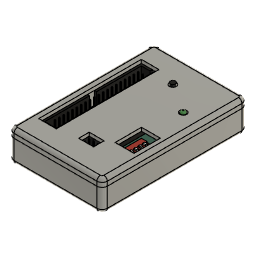
PETDiag_Clip v4 (Autodesk Fusion 360 design; units mm, degrees)
Autodesk Fusion 360 part; units mm, degrees
note: some values were not read from the file. Set by a fixed rule: which sketch regions a step uses.
(part 1 of 2)
sketch "dxf" plane through (0, 0, 0) normal (0, 0, 1) x (1, 0, 0) in component "PCB"
  line L0 (47, 0) -> (47, 77)
  line L1 (0, 77) -> (0, 0)
  line L2 (0, 0) -> (47, 0)
  line L3 (47, 77) -> (0, 77)
  line L4 (43.3388, 35.4013) -> (43.0213, 35.0838)
  line L5 (38.8938, 35.4013) -> (43.3388, 35.4013)
  line L6 (38.8938, 35.4013) -> (39.2112, 35.0838)
  line L7 (38.8938, 35.4013) -> (39.2112, 35.7188)
  line L8 (43.3388, 35.4013) -> (43.0213, 35.7188)
  line L9 (20.9118, 60.9092) -> (21.4311, 60.9092)
  arc A0 (22.4081, 60.8118) -> (22.116, 60.9092) centre (22.116, 60.4224) ccw
  line L10 (21.4311, 59.7408) -> (20.9118, 59.7408)
  line L11 (23.8432, 60.9092) -> (24.4923, 60.9092)
  line L12 (23.4885, 59.7408) -> (22.9692, 59.7408)
  line L13 (22.9692, 60.3899) -> (23.3587, 60.3899)
  arc A1 (22.2134, 59.7408) -> (22.473, 60.0004) centre (22.2134, 60.0004) ccw
  line L14 (22.9692, 59.7408) -> (22.9692, 60.9092)
  arc A2 (21.8564, 60.6496) -> (21.9862, 60.4224) centre (22.1201, 60.6496) ccw
  line L15 (19.685, 61.1124) -> (24.5431, 61.1124)
  line L16 (19.7358, 59.7408) -> (19.7358, 60.9092)
  arc A3 (21.8239, 59.9031) -> (22.2134, 59.7408) centre (22.2134, 60.2893) ccw
  arc A4 (22.473, 60.0004) -> (22.3432, 60.2276) centre (22.2093, 60.0004) ccw
  arc A5 (22.116, 60.9092) -> (21.8564, 60.6496) centre (22.116, 60.6496) ccw
  line L17 (19.7358, 60.9092) -> (20.0604, 60.9092)
  line L18 (24.1678, 59.7408) -> (24.1678, 60.9092)
  line L19 (22.9692, 60.9092) -> (23.4885, 60.9092)
  line L20 (20.9118, 59.7408) -> (20.9118, 60.9092)
  arc A6 (20.0604, 60.26) -> (20.0604, 60.9092) centre (20.0604, 60.5846) ccw
  line L21 (20.0604, 60.2601) -> (19.7358, 60.2601)
  line L22 (20.9118, 60.3899) -> (21.3013, 60.3899)
  line L23 (22.3432, 60.2276) -> (21.9862, 60.4224)
  line L24 (20.3849, 59.7408) -> (20.1253, 60.2601)
  line L25 (38.0492, 35.9855) -> (38.0492, 34.8171)
  line L26 (44.0246, 34.8171) -> (44.5438, 34.8171)
  line L27 (37.4001, 34.8171) -> (37.4001, 35.9855)
  line L28 (44.0246, 35.9855) -> (44.0246, 34.8171)
  line L29 (37.4001, 35.4662) -> (38.0492, 35.4662)
  line L30 (1.7462, 63.1975) -> (1.7462, 63.3563)
  arc A7 (16.383, 5.334) -> (16.383, 7.366) centre (16.383, 6.35) ccw
  arc A8 (23.3363, 18.542) -> (20.7963, 18.542) centre (22.0663, 18.542) ccw
  circle A9 centre (5, 72) radius 3.1789
  line L31 (1.7462, 63.3563) -> (1.7462, 63.515)
  line L32 (1.7462, 40.8138) -> (1.7462, 62.0863)
  line L33 (1.7462, 63.6738) -> (1.7462, 67.96)
  line L34 (28.6703, 53.848) -> (15.4623, 53.848)
  line L35 (1.7462, 62.0863) -> (1.7462, 62.4038)
  line L36 (8.0963, 67.96) -> (9.525, 67.96)
  line L37 (1.7462, 63.515) -> (1.7462, 63.6738)
  line L38 (10.9538, 9.54) -> (9.525, 9.54)
  line L39 (23.3362, 18.542) -> (28.6703, 18.542)
  circle A10 centre (5, 5) radius 3.1789
  line L40 (15.4623, 18.542) -> (15.4623, 53.848)
  line L41 (1.7462, 67.96) -> (8.0963, 67.96)
  line L42 (16.383, 3.302) -> (35.687, 3.302)
  line L43 (1.7462, 62.88) -> (1.7462, 63.0388)
  line L44 (9.525, 9.54) -> (8.0963, 9.54)
  line L45 (1.7462, 62.7213) -> (1.7462, 62.88)
  line L46 (35.687, 9.398) -> (16.383, 9.398)
  line L47 (8.0963, 10.3337) -> (8.0963, 9.54)
  line L48 (2.54, 40.8138) -> (1.7462, 40.8138)
  line L49 (10.16, 67.1663) -> (10.16, 10.3337)
  line L50 (1.7462, 9.54) -> (1.7462, 36.6862)
  line L51 (3.0162, 10.81) -> (2.54, 10.3337)
  line L52 (28.6703, 18.542) -> (28.6703, 53.848)
  line L53 (7.366, 62.626) -> (7.874, 62.626)
  line L54 (8.0963, 10.3337) -> (2.54, 10.3337)
  line L55 (9.525, 66.69) -> (9.6838, 66.69)
  line L56 (9.525, 10.81) -> (8.0963, 10.81)
  line L57 (3.0162, 40.8138) -> (3.0162, 66.69)
  line L58 (1.7462, 36.6862) -> (1.7462, 40.8138)
  line L59 (8.0963, 66.69) -> (8.0963, 67.1663)
  arc A11 (10.9538, 38.2738) -> (10.9538, 39.385) centre (10.9538, 38.8294) ccw
  line L60 (15.4623, 18.542) -> (20.7963, 18.542)
  line L61 (1.7462, 62.5625) -> (1.7462, 62.7213)
  line L62 (1.7462, 63.1975) -> (1.7462, 63.0388)
  line L63 (2.54, 36.6862) -> (1.7462, 36.6862)
  line L64 (9.6838, 10.81) -> (9.525, 10.81)
  line L65 (8.0963, 9.54) -> (1.7462, 9.54)
  line L66 (3.0162, 36.6862) -> (2.54, 36.6862)
  line L67 (9.6838, 66.69) -> (9.6838, 10.81)
  line L68 (3.0162, 10.81) -> (3.0162, 36.6862)
  line L69 (1.7462, 62.5625) -> (1.7463, 62.5625)
  line L70 (8.0963, 10.81) -> (3.0162, 10.81)
  circle A12 centre (5, 5) radius 1.7463
  circle A13 centre (42, 72) radius 1.7463
  line L71 (35.687, 9.398) -> (35.687, 3.302)
  line L72 (9.525, 10.3337) -> (10.16, 10.3337)
  line L73 (16.383, 9.398) -> (16.383, 7.366)
  circle A14 centre (42, 5) radius 1.7463
  line L74 (4.826, 62.626) -> (5.334, 62.626)
  line L75 (9.525, 10.81) -> (9.525, 10.3337)
  line L76 (9.525, 66.69) -> (9.525, 67.1663)
  line L77 (16.383, 3.302) -> (16.383, 5.334)
  arc A15 (10.9538, 65.42) -> (10.9538, 66.69) centre (10.9538, 66.055) ccw
  line L78 (8.0963, 67.1663) -> (8.0963, 67.96)
  line L79 (9.525, 10.3337) -> (9.525, 9.54)
  line L80 (5.334, 62.626) -> (5.334, 63.134)
  line L81 (9.525, 67.1663) -> (9.525, 67.96)
  line L82 (3.0162, 66.69) -> (8.0963, 66.69)
  line L83 (10.16, 67.1663) -> (9.6838, 66.69)
  line L84 (1.7462, 62.4038) -> (1.7462, 62.5625)
  line L85 (10.9538, 67.96) -> (10.9538, 9.54)
  circle A16 centre (5, 72) radius 1.7463
  line L86 (2.2225, 62.7213) -> (2.2224, 62.7213)
  line L87 (10.16, 67.1663) -> (9.525, 67.1663)
  circle A17 centre (42, 72) radius 3.1789
  line L88 (2.54, 62.88) -> (2.5399, 62.88)
  line L89 (8.0963, 67.1663) -> (2.54, 67.1663)
  circle A18 centre (42, 5) radius 3.1789
  line L90 (5.334, 55.006) -> (5.334, 55.514)
  line L91 (7.366, 57.546) -> (7.874, 57.546)
  line L92 (7.366, 52.974) -> (7.366, 52.466)
  line L93 (7.874, 52.466) -> (7.874, 52.974)
  line L94 (4.826, 58.054) -> (4.826, 57.546)
  line L95 (5.334, 55.514) -> (4.826, 55.514)
  line L96 (5.334, 60.086) -> (5.334, 60.594)
  line L97 (4.826, 57.546) -> (5.334, 57.546)
  line L98 (7.874, 60.594) -> (7.366, 60.594)
  line L99 (4.826, 63.134) -> (4.826, 62.626)
  line L100 (7.874, 63.134) -> (7.366, 63.134)
  line L101 (7.366, 52.466) -> (7.874, 52.466)
  line L102 (7.874, 55.514) -> (7.366, 55.514)
  line L103 (4.826, 55.514) -> (4.826, 55.006)
  line L104 (4.826, 60.086) -> (5.334, 60.086)
  line L105 (2.54, 36.6862) -> (2.54, 10.3337)
  line L106 (4.826, 49.926) -> (5.334, 49.926)
  line L107 (7.874, 49.926) -> (7.874, 50.434)
  line L108 (4.826, 52.466) -> (5.334, 52.466)
  line L109 (7.366, 58.054) -> (7.366, 57.546)
  line L110 (7.874, 52.974) -> (7.366, 52.974)
  line L111 (3.0162, 36.6862) -> (3.0162, 40.8138)
  line L112 (9.6838, 10.81) -> (10.16, 10.3337)
  line L113 (5.334, 47.894) -> (4.826, 47.894)
  line L114 (7.366, 49.926) -> (7.874, 49.926)
  line L115 (9.525, 67.96) -> (10.9538, 67.96)
  line L116 (2.54, 62.88) -> (2.54, 67.1663)
  line L117 (7.366, 50.434) -> (7.366, 49.926)
  line L118 (5.334, 52.974) -> (4.826, 52.974)
  line L119 (7.366, 44.846) -> (7.874, 44.846)
  line L120 (7.874, 57.546) -> (7.874, 58.054)
  line L121 (2.54, 40.8138) -> (2.54, 62.88)
  line L122 (4.826, 60.594) -> (4.826, 60.086)
  line L123 (7.874, 55.006) -> (7.874, 55.514)
  line L124 (7.366, 55.514) -> (7.366, 55.006)
  line L125 (4.826, 50.434) -> (4.826, 49.926)
  line L126 (7.874, 50.434) -> (7.366, 50.434)
  line L127 (5.334, 50.434) -> (4.826, 50.434)
  line L128 (5.334, 58.054) -> (4.826, 58.054)
  line L129 (7.366, 45.354) -> (7.366, 44.846)
  arc A19 (10.9538, 10.81) -> (10.9538, 12.08) centre (10.9538, 11.445) ccw
  line L130 (5.334, 49.926) -> (5.334, 50.434)
  line L131 (4.826, 47.386) -> (5.334, 47.386)
  line L132 (5.334, 47.386) -> (5.334, 47.894)
  line L133 (4.826, 55.006) -> (5.334, 55.006)
  line L134 (7.366, 60.594) -> (7.366, 60.086)
  line L135 (3.0162, 40.8138) -> (2.54, 40.8138)
  line L136 (5.334, 63.134) -> (4.826, 63.134)
  line L137 (8.0963, 10.81) -> (8.0963, 10.3337)
  line L138 (7.874, 62.626) -> (7.874, 63.134)
  line L139 (2.54, 67.1663) -> (3.0162, 66.69)
  line L140 (8.0963, 66.69) -> (9.525, 66.69)
  line L141 (7.874, 60.086) -> (7.874, 60.594)
  line L142 (7.366, 63.134) -> (7.366, 62.626)
  line L143 (7.366, 47.386) -> (7.874, 47.386)
  line L144 (5.334, 60.594) -> (4.826, 60.594)
  line L145 (5.334, 52.466) -> (5.334, 52.974)
  line L146 (7.874, 47.894) -> (7.366, 47.894)
  line L147 (7.874, 47.386) -> (7.874, 47.894)
  line L148 (4.826, 47.894) -> (4.826, 47.386)
  line L149 (7.874, 58.054) -> (7.366, 58.054)
  line L150 (7.366, 34.686) -> (7.874, 34.686)
  line L151 (7.366, 32.654) -> (7.366, 32.146)
  line L152 (4.826, 32.654) -> (4.826, 32.146)
  line L153 (7.874, 32.654) -> (7.366, 32.654)
  line L154 (7.366, 47.894) -> (7.366, 47.386)
  line L155 (7.366, 37.734) -> (7.366, 37.226)
  line L156 (4.826, 39.766) -> (5.334, 39.766)
  line L157 (5.334, 45.354) -> (4.826, 45.354)
  line L158 (7.874, 40.274) -> (7.366, 40.274)
  line L159 (7.874, 30.114) -> (7.366, 30.114)
  line L160 (7.874, 42.306) -> (7.874, 42.814)
  line L161 (7.366, 60.086) -> (7.874, 60.086)
  line L162 (7.874, 42.814) -> (7.366, 42.814)
  line L163 (5.334, 32.654) -> (4.826, 32.654)
  line L164 (5.334, 37.734) -> (4.826, 37.734)
  line L165 (5.334, 42.814) -> (4.826, 42.814)
  line L166 (5.334, 40.274) -> (4.826, 40.274)
  line L167 (7.366, 55.006) -> (7.874, 55.006)
  line L168 (4.826, 42.814) -> (4.826, 42.306)
  line L169 (5.334, 42.306) -> (5.334, 42.814)
  line L170 (7.874, 44.846) -> (7.874, 45.354)
  line L171 (7.874, 32.146) -> (7.874, 32.654)
  line L172 (7.874, 45.354) -> (7.366, 45.354)
  line L173 (7.874, 34.686) -> (7.874, 35.194)
  line L174 (5.334, 39.766) -> (5.334, 40.274)
  line L175 (4.826, 44.846) -> (5.334, 44.846)
  line L176 (7.366, 35.194) -> (7.366, 34.686)
  line L177 (4.826, 40.274) -> (4.826, 39.766)
  line L178 (7.366, 32.146) -> (7.874, 32.146)
  line L179 (5.334, 25.034) -> (4.826, 25.034)
  line L180 (4.826, 19.446) -> (5.334, 19.446)
  line L181 (4.826, 32.146) -> (5.334, 32.146)
  line L182 (5.334, 29.606) -> (5.334, 30.114)
  line L183 (5.334, 19.954) -> (4.826, 19.954)
  line L184 (4.826, 25.034) -> (4.826, 24.526)
  line L185 (4.826, 34.686) -> (5.334, 34.686)
  line L186 (4.826, 35.194) -> (4.826, 34.686)
  line L187 (4.826, 37.226) -> (5.334, 37.226)
  line L188 (7.874, 37.226) -> (7.874, 37.734)
  line L189 (4.826, 45.354) -> (4.826, 44.846)
  line L190 (7.874, 29.606) -> (7.874, 30.114)
  line L191 (7.366, 37.226) -> (7.874, 37.226)
  line L192 (7.366, 42.306) -> (7.874, 42.306)
  line L193 (7.874, 39.766) -> (7.874, 40.274)
  line L194 (7.366, 29.606) -> (7.874, 29.606)
  line L195 (5.334, 37.226) -> (5.334, 37.734)
  line L196 (7.366, 40.274) -> (7.366, 39.766)
  line L197 (4.826, 19.954) -> (4.826, 19.446)
  line L198 (4.826, 21.986) -> (5.334, 21.986)
  line L199 (7.366, 30.114) -> (7.366, 29.606)
  line L200 (5.334, 27.574) -> (4.826, 27.574)
  line L201 (5.334, 57.546) -> (5.334, 58.054)
  line L202 (4.826, 52.974) -> (4.826, 52.466)
  line L203 (5.334, 32.146) -> (5.334, 32.654)
  line L204 (7.874, 35.194) -> (7.366, 35.194)
  line L205 (5.334, 44.846) -> (5.334, 45.354)
  line L206 (7.366, 39.766) -> (7.874, 39.766)
  line L207 (7.366, 42.814) -> (7.366, 42.306)
  line L208 (4.826, 37.734) -> (4.826, 37.226)
  line L209 (7.874, 37.734) -> (7.366, 37.734)
  line L210 (4.826, 30.114) -> (4.826, 29.606)
  line L211 (5.334, 34.686) -> (5.334, 35.194)
  line L212 (4.826, 42.306) -> (5.334, 42.306)
  line L213 (5.334, 35.194) -> (4.826, 35.194)
  line L214 (5.334, 22.494) -> (4.826, 22.494)
  line L215 (34.29, 53.975) -> (33.02, 53.975)
  line L216 (28.2575, 15.7163) -> (28.2575, 11.9063)
  line L217 (34.29, 48.895) -> (33.02, 48.895)
  line L218 (25.0825, 11.2713) -> (25.7175, 11.9063)
  line L219 (30.7975, 15.7163) -> (30.7975, 11.9063)
  line L220 (7.874, 19.954) -> (7.366, 19.954)
  line L221 (5.334, 21.986) -> (5.334, 22.494)
  line L222 (23.8125, 16.3513) -> (25.0825, 16.3513)
  line L223 (7.366, 25.034) -> (7.366, 24.526)
  line L224 (5.334, 19.446) -> (5.334, 19.954)
  line L225 (7.366, 16.906) -> (7.874, 16.906)
  line L226 (26.3525, 11.2713) -> (27.6225, 11.2713)
  line L227 (25.7175, 15.7163) -> (25.7175, 11.9063)
  line L228 (5.334, 16.906) -> (5.334, 17.414)
  line L229 (4.826, 17.414) -> (4.826, 16.906)
  line L230 (26.3525, 16.3513) -> (27.6225, 16.3513)
  line L231 (28.2575, 15.7163) -> (28.8925, 16.3513)
  line L232 (7.874, 24.526) -> (7.874, 25.034)
  line L233 (4.826, 14.874) -> (4.826, 14.366)
  line L234 (7.874, 19.446) -> (7.874, 19.954)
  line L235 (7.874, 25.034) -> (7.366, 25.034)
  line L236 (7.874, 27.066) -> (7.874, 27.574)
  line L237 (7.366, 27.574) -> (7.366, 27.066)
  line L238 (7.874, 27.574) -> (7.366, 27.574)
  line L239 (23.1775, 11.9063) -> (23.1775, 15.7163)
  line L240 (7.874, 14.874) -> (7.366, 14.874)
  line L241 (32.385, 52.07) -> (32.385, 53.975)
  line L242 (7.366, 19.446) -> (7.874, 19.446)
  line L243 (5.334, 30.114) -> (4.826, 30.114)
  line L244 (7.366, 19.954) -> (7.366, 19.446)
  line L245 (4.826, 16.906) -> (5.334, 16.906)
  line L246 (7.366, 21.986) -> (7.874, 21.986)
  line L247 (25.7175, 11.9063) -> (26.3525, 11.2713)
  line L248 (32.385, 49.53) -> (32.385, 50.8)
  line L249 (33.02, 53.975) -> (32.385, 53.975)
  line L250 (34.925, 50.8) -> (34.925, 49.53)
  line L251 (4.826, 22.494) -> (4.826, 21.986)
  line L252 (7.874, 14.366) -> (7.874, 14.874)
  line L253 (5.334, 14.366) -> (5.334, 14.874)
  line L254 (5.334, 27.066) -> (5.334, 27.574)
  line L255 (4.826, 27.066) -> (5.334, 27.066)
  line L256 (5.334, 14.874) -> (4.826, 14.874)
  line L257 (4.826, 27.574) -> (4.826, 27.066)
  line L258 (27.6225, 11.2713) -> (28.2575, 11.9063)
  line L259 (7.366, 14.874) -> (7.366, 14.366)
  line L260 (7.874, 17.414) -> (7.366, 17.414)
  line L261 (7.366, 22.494) -> (7.366, 21.986)
  line L262 (7.874, 22.494) -> (7.366, 22.494)
  line L263 (5.334, 17.414) -> (4.826, 17.414)
  line L264 (5.334, 24.526) -> (5.334, 25.034)
  line L265 (7.874, 21.986) -> (7.874, 22.494)
  line L266 (7.366, 24.526) -> (7.874, 24.526)
  line L267 (7.366, 27.066) -> (7.874, 27.066)
  line L268 (7.366, 17.414) -> (7.366, 16.906)
  line L269 (4.826, 24.526) -> (5.334, 24.526)
  line L270 (4.826, 14.366) -> (5.334, 14.366)
  line L271 (7.366, 14.366) -> (7.874, 14.366)
  line L272 (4.826, 29.606) -> (5.334, 29.606)
  line L273 (7.874, 16.906) -> (7.874, 17.414)
  line L274 (34.925, 52.07) -> (34.6075, 51.7525)
  line L275 (27.6225, 16.3513) -> (28.2575, 15.7163)
  line L276 (34.6075, 51.1175) -> (34.925, 50.8)
  line L277 (34.925, 53.34) -> (34.925, 52.07)
  circle A20 centre (23, 65) radius 1.75
  arc A21 (25.45, 63.25) -> (25.45, 62.45) centre (25.15, 62.85) ccw
  line L278 (34.925, 53.34) -> (34.29, 53.975)
  line L279 (25.7175, 15.7163) -> (26.3525, 16.3513)
  line L280 (32.7025, 51.7525) -> (32.385, 52.07)
  line L281 (30.1625, 11.2713) -> (30.7975, 11.9063)
  line L282 (45.7518, 33.9408) -> (42.4498, 33.9408)
  line L283 (26, 66.45) -> (26, 63.6)
  line L284 (23.1775, 11.9063) -> (23.1775, 11.2713)
  line L285 (30.1625, 16.3513) -> (30.7975, 15.7163)
  line L286 (25.0825, 16.3513) -> (25.7175, 15.7163)
  line L287 (28.8925, 16.3513) -> (30.1625, 16.3513)
  line L288 (32.385, 50.8) -> (32.7025, 51.1175)
  line L289 (23.1775, 11.2713) -> (25.0825, 11.2713)
  line L290 (28.8925, 11.2713) -> (30.1625, 11.2713)
  arc A22 (41.5, 54.8) -> (38.5, 54.8) centre (40, 54) ccw
  arc A23 (20.55, 62.45) -> (20.5, 63.2) centre (20.8502, 62.8467) ccw
  circle A24 centre (23, 65) radius 1.4
  line L291 (28.2575, 11.9063) -> (28.8925, 11.2713)
  line L292 (23.1775, 15.7163) -> (23.8125, 16.3513)
  line L293 (25.4, 62) -> (20.25, 62)
  line L294 (20, 63.55) -> (20, 66.45)
  arc A25 (20.55, 66.75) -> (20.5, 67.5) centre (20.8502, 67.1467) ccw
  line L295 (33.02, 48.895) -> (32.385, 49.53)
  arc A26 (41.5, 54.8) -> (38.5, 54.8) centre (40, 54) ccw
  arc A27 (38.5, 53.2) -> (41.5, 53.2) centre (40, 54) ccw
  line L296 (34.925, 49.53) -> (34.29, 48.895)
  arc A28 (38.5, 53.2) -> (41.5, 53.2) centre (40, 54) ccw
  line L297 (39.1478, 33.4327) -> (42.4498, 33.4327)
  line L298 (20.25, 68) -> (25.75, 68)
  line L299 (41.6878, 32.6707) -> (38.8938, 32.6707)
  line L300 (39.1478, 33.9408) -> (35.8458, 33.9408)
  line L301 (42.4498, 32.6707) -> (42.7037, 32.6707)
  line L302 (35.8458, 19.7168) -> (39.1478, 19.7168)
  line L303 (38.8938, 23.5267) -> (41.6878, 23.5267)
  line L304 (42.4498, 19.7168) -> (45.7518, 19.7168)
  line L305 (41.6878, 25.0508) -> (38.8938, 25.0508)
  line L306 (38.8938, 23.5267) -> (38.8938, 25.0508)
  line L307 (42.7037, 31.1468) -> (42.4498, 31.1468)
  line L308 (40.7988, 24.7968) -> (39.1478, 24.7968)
  line L309 (42.7037, 28.8608) -> (42.7037, 28.6068)
  line L310 (42.7037, 23.5267) -> (42.4498, 23.5267)
  line L311 (42.7037, 25.0508) -> (42.7037, 24.7968)
  line L312 (38.8938, 20.9868) -> (41.6878, 20.9868)
  line L313 (40.7988, 29.8768) -> (39.1478, 29.8768)
  line L314 (42.4498, 30.1308) -> (42.7037, 30.1308)
  line L315 (38.8938, 31.1468) -> (41.6878, 31.1468)
  line L316 (40.7988, 21.2408) -> (39.1478, 21.2408)
  line L317 (40.7988, 22.2568) -> (39.1478, 22.2568)
  line L318 (40.7988, 26.3208) -> (39.1478, 26.3208)
  line L319 (42.4498, 33.4327) -> (42.4498, 33.9408)
  line L320 (42.7037, 31.4008) -> (42.7037, 31.1468)
  line L321 (38.8938, 28.6068) -> (38.8938, 30.1308)
  line L322 (42.7037, 26.3208) -> (42.7037, 26.0668)
  line L323 (40.7988, 28.8608) -> (39.1478, 28.8608)
  line L324 (40.7988, 27.3368) -> (39.1478, 27.3368)
  line L325 (39.1478, 29.8768) -> (39.1478, 28.8608)
  line L326 (42.4498, 20.2248) -> (39.1478, 20.2248)
  line L327 (41.6878, 30.1308) -> (38.8938, 30.1308)
  line L328 (38.8938, 28.6068) -> (41.6878, 28.6068)
  line L329 (39.1478, 33.9408) -> (39.1478, 33.4327)
  line L330 (42.7037, 27.5907) -> (42.7037, 27.3368)
  line L331 (38.8938, 26.0668) -> (38.8938, 27.5907)
  line L332 (39.1478, 20.2248) -> (39.1478, 19.7168)
  line L333 (42.7037, 30.1308) -> (42.7037, 29.8768)
  arc A29 (25.45, 67.55) -> (25.5, 66.8) centre (25.1498, 67.1533) ccw
  line L334 (42.7037, 32.6707) -> (42.7037, 32.4168)
  line L335 (39.1478, 19.7168) -> (42.4498, 19.7168)
  line L336 (35.8458, 33.9408) -> (35.8458, 19.7168)
  line L337 (40.7988, 32.4168) -> (39.1478, 32.4168)
  line L338 (42.4498, 27.5907) -> (42.7037, 27.5907)
  line L339 (42.7037, 23.7808) -> (42.7037, 23.5267)
  line L340 (42.4498, 19.7168) -> (42.4498, 20.2248)
  line L341 (41.6878, 22.5108) -> (38.8938, 22.5108)
  line L342 (40.7988, 31.4008) -> (39.1478, 31.4008)
  line L343 (41.6878, 27.5907) -> (38.8938, 27.5907)
  line L344 (38.8938, 20.9868) -> (38.8938, 22.5108)
  line L345 (38.8938, 31.1468) -> (38.8938, 32.6707)
  line L346 (42.4498, 25.0508) -> (42.7037, 25.0508)
  line L347 (45.7518, 19.7168) -> (45.7518, 33.9408)
  line L348 (42.7037, 28.6068) -> (42.4498, 28.6068)
  line L349 (38.8938, 26.0668) -> (41.6878, 26.0668)
  line L350 (42.4498, 33.9408) -> (39.1478, 33.9408)
  line L351 (42.7037, 26.0668) -> (42.4498, 26.0668)
  line L352 (40.7988, 23.7808) -> (39.1478, 23.7808)
  line L353 (40.7988, 22.2568) -> (40.4178, 22.2568)
  line L354 (39.7828, 27.3368) -> (39.7828, 26.3208)
  line L355 (40.7988, 28.8608) -> (40.7988, 29.8768)
  line L356 (40.7988, 31.4008) -> (40.7988, 32.4168)
  line L357 (39.5288, 32.4168) -> (39.1478, 32.4168)
  line L358 (39.5288, 21.2408) -> (39.5288, 22.2568)
  line L359 (39.1478, 26.3208) -> (39.5288, 26.3208)
  line L360 (40.4178, 23.7808) -> (40.7988, 23.7808)
  line L361 (39.1478, 23.7808) -> (39.5288, 23.7808)
  line L362 (39.7828, 32.4168) -> (39.7828, 31.4008)
  line L363 (40.4178, 24.7968) -> (40.4178, 23.7808)
  line L364 (39.5288, 23.7808) -> (39.5288, 24.7968)
  line L365 (39.1478, 31.4008) -> (39.5288, 31.4008)
  line L366 (39.5288, 26.3208) -> (39.5288, 27.3368)
  line L367 (39.7828, 21.2408) -> (40.1638, 21.2408)
  line L368 (39.7828, 26.3208) -> (40.1638, 26.3208)
  line L369 (40.1638, 23.7808) -> (40.1638, 24.7968)
  line L370 (39.1478, 22.2568) -> (39.1478, 21.2408)
  line L371 (40.4178, 28.8608) -> (40.7988, 28.8608)
  line L372 (42.7037, 20.9868) -> (42.4498, 20.9868)
  line L373 (40.4178, 22.2568) -> (40.4178, 21.2408)
  line L374 (40.1638, 27.3368) -> (39.7828, 27.3368)
  line L375 (39.7828, 23.7808) -> (40.1638, 23.7808)
  line L376 (39.7828, 28.8608) -> (40.1638, 28.8608)
  line L377 (39.1478, 24.7968) -> (39.1478, 23.7808)
  line L378 (39.1478, 21.2408) -> (39.5288, 21.2408)
  line L379 (40.1638, 22.2568) -> (39.7828, 22.2568)
  line L380 (42.7037, 22.5108) -> (42.7037, 22.2568)
  line L381 (40.4178, 29.8768) -> (40.4178, 28.8608)
  line L382 (39.5288, 22.2568) -> (39.1478, 22.2568)
  line L383 (40.7988, 32.4168) -> (40.4178, 32.4168)
  line L384 (40.7988, 21.2408) -> (40.7988, 22.2568)
  line L385 (39.5288, 31.4008) -> (39.5288, 32.4168)
  line L386 (40.7988, 23.7808) -> (40.7988, 24.7968)
  line L387 (40.4178, 21.2408) -> (40.7988, 21.2408)
  line L388 (40.1638, 29.8768) -> (39.7828, 29.8768)
  line L389 (40.7988, 26.3208) -> (40.7988, 27.3368)
  line L390 (39.7828, 31.4008) -> (40.1638, 31.4008)
  line L391 (40.4178, 32.4168) -> (40.4178, 31.4008)
  line L392 (40.1638, 21.2408) -> (40.1638, 22.2568)
  line L393 (40.1638, 31.4008) -> (40.1638, 32.4168)
  line L394 (40.4178, 31.4008) -> (40.7988, 31.4008)
  line L395 (40.1638, 32.4168) -> (39.7828, 32.4168)
  line L396 (40.7988, 27.3368) -> (40.4178, 27.3368)
  line L397 (39.7828, 29.8768) -> (39.7828, 28.8608)
  line L398 (39.5288, 28.8608) -> (39.5288, 29.8768)
  line L399 (39.1478, 27.3368) -> (39.1478, 26.3208)
  line L400 (39.1478, 28.8608) -> (39.5288, 28.8608)
  line L401 (40.1638, 28.8608) -> (40.1638, 29.8768)
  line L402 (39.5288, 24.7968) -> (39.1478, 24.7968)
  line L403 (42.7037, 21.2408) -> (42.7037, 20.9868)
  line L404 (39.5288, 27.3368) -> (39.1478, 27.3368)
  line L405 (39.1478, 32.4168) -> (39.1478, 31.4008)
  line L406 (42.4498, 22.5108) -> (42.7037, 22.5108)
  line L407 (40.7988, 29.8768) -> (40.4178, 29.8768)
  line L408 (39.7828, 22.2568) -> (39.7828, 21.2408)
  line L409 (40.4178, 26.3208) -> (40.7988, 26.3208)
  line L410 (40.4178, 27.3368) -> (40.4178, 26.3208)
  line L411 (40.7988, 24.7968) -> (40.4178, 24.7968)
  line L412 (39.7828, 24.7968) -> (39.7828, 23.7808)
  line L413 (40.1638, 26.3208) -> (40.1638, 27.3368)
  line L414 (40.1638, 24.7968) -> (39.7828, 24.7968)
  line L415 (39.5288, 29.8768) -> (39.1478, 29.8768)
  line L416 (24.7015, 12.2872) -> (24.7015, 12.7952)
  line L417 (24.7015, 12.7952) -> (24.1935, 12.7952)
  line L418 (33.401, 52.959) -> (33.401, 52.451)
  line L419 (34.6075, 51.7525) -> (34.29, 51.435)
  line L420 (34.29, 51.435) -> (33.02, 51.435)
  line L421 (24.1935, 12.7952) -> (24.1935, 12.2872)
  line L422 (33.909, 52.451) -> (33.909, 52.959)
  line L423 (24.7015, 14.8273) -> (24.7015, 15.3353)
  line L424 (26.7335, 12.2872) -> (27.2415, 12.2872)
  line L425 (29.2735, 15.3353) -> (29.2735, 14.8273)
  line L426 (33.909, 52.959) -> (33.401, 52.959)
  line L427 (26.7335, 12.7952) -> (26.7335, 12.2872)
  line L428 (29.7815, 12.2872) -> (29.7815, 12.7952)
  line L429 (32.7025, 51.1175) -> (33.02, 51.435)
  line L430 (33.401, 50.419) -> (33.401, 49.911)
  line L431 (33.909, 50.419) -> (33.401, 50.419)
  line L432 (33.02, 51.435) -> (32.7025, 51.7525)
  line L433 (34.29, 51.435) -> (34.6075, 51.1175)
  line L434 (33.401, 52.451) -> (33.909, 52.451)
  line L435 (33.909, 49.911) -> (33.909, 50.419)
  line L436 (33.401, 49.911) -> (33.909, 49.911)
  line L437 (24.1935, 12.2872) -> (24.7015, 12.2872)
  line L438 (27.2415, 14.8273) -> (27.2415, 15.3353)
  line L439 (25.75, 68) -> (25.8, 68)
  line L440 (20, 63.1) -> (19.5, 63.1)
  line L441 (19.5, 63.1) -> (19.5, 62.4)
  line L442 (26.5, 63.1) -> (26, 63.1)
  arc A30 (25.5, 66.8) -> (25.45, 67.55) centre (25.1498, 67.1533) ccw
  line L443 (26, 67.8) -> (26, 66.45)
  line L444 (26, 63.1) -> (26, 62.4)
  arc A31 (25.45, 62.45) -> (25.45, 63.25) centre (25.15, 62.85) ccw
  line L445 (26, 67.6) -> (26, 66.9)
  line L446 (20, 62.2) -> (20, 63.55)
  line L447 (25.8, 62) -> (25.4, 62)
  line L448 (26, 66.9) -> (26.5, 66.9)
  arc A32 (20.5, 63.2) -> (20.55, 62.45) centre (20.8502, 62.8467) ccw
  arc A33 (20.2, 68) -> (20, 67.8) centre (20.2, 67.8) ccw
  arc A34 (20, 62.2) -> (20.2, 62) centre (20.2, 62.2) ccw
  line L449 (29.7815, 12.7952) -> (29.2735, 12.7952)
  line L450 (19.5, 66.9) -> (20, 66.9)
  line L451 (26, 62.4) -> (26.5, 62.4)
  line L452 (26.5, 62.4) -> (26.5, 63.1)
  arc A35 (20.5, 67.5) -> (20.55, 66.75) centre (20.8502, 67.1467) ccw
  line L453 (27.2415, 12.2872) -> (27.2415, 12.7952)
  line L454 (24.7015, 15.3353) -> (24.1935, 15.3353)
  line L455 (19.5, 62.4) -> (20, 62.4)
  line L456 (42.7037, 27.3368) -> (42.7037, 26.3208)
  circle A36 centre (40, 54) radius 1.5
  line L457 (29.2735, 14.8273) -> (29.7815, 14.8273)
  line L458 (42.4498, 28.6068) -> (41.6878, 28.6068)
  line L459 (20, 66.9) -> (20, 67.6)
  line L460 (42.7037, 24.7968) -> (42.7037, 23.7808)
  line L461 (20.25, 62) -> (20.2, 62)
  line L462 (42.4498, 30.1308) -> (41.6878, 30.1308)
  line L463 (20, 66.45) -> (20, 67.8)
  line L464 (26.5, 67.6) -> (26, 67.6)
  line L465 (42.4498, 31.1468) -> (41.6878, 31.1468)
  line L466 (19.5, 67.6) -> (19.5, 66.9)
  line L467 (42.4498, 23.5267) -> (41.6878, 23.5267)
  line L468 (42.4498, 27.5907) -> (41.6878, 27.5907)
  arc A37 (41.5, 53.2) -> (41.5, 54.8) centre (40, 54) ccw
  line L469 (27.2415, 12.7952) -> (26.7335, 12.7952)
  line L470 (29.7815, 14.8273) -> (29.7815, 15.3353)
  line L471 (26.7335, 15.3353) -> (26.7335, 14.8273)
  line L472 (29.2735, 12.7952) -> (29.2735, 12.2872)
  line L473 (20, 62.4) -> (20, 63.1)
  line L474 (20, 67.6) -> (19.5, 67.6)
  line L475 (26, 63.6) -> (26, 62.2)
  arc A38 (25.8, 62) -> (26, 62.2) centre (25.8, 62.2) ccw
  line L476 (24.1935, 15.3353) -> (24.1935, 14.8273)
  line L477 (26.7335, 14.8273) -> (27.2415, 14.8273)
  line L478 (29.2735, 12.2872) -> (29.7815, 12.2872)
  line L479 (27.2415, 15.3353) -> (26.7335, 15.3353)
  line L480 (29.7815, 15.3353) -> (29.2735, 15.3353)
  line L481 (20.2, 68) -> (20.25, 68)
  line L482 (26.5, 66.9) -> (26.5, 67.6)
  line L483 (24.1935, 14.8273) -> (24.7015, 14.8273)
  line L484 (38.5, 53.2) -> (38.5, 54.8)
  arc A39 (26, 67.8) -> (25.8, 68) centre (25.8, 67.8) ccw
  line L485 (36.6713, 21.4171) -> (36.6713, 22.1933)
  line L486 (37.7578, 23.9571) -> (37.7578, 24.7333)
  line L487 (42.4498, 20.9868) -> (41.6878, 20.9868)
  line L488 (37.4474, 24.5004) -> (38.0682, 24.5004)
  line L489 (38.0682, 29.0371) -> (38.0682, 29.8133)
  arc A40 (37.6026, 22.1932) -> (37.2922, 21.8828) centre (37.6026, 21.8828) ccw
  line L490 (43.7903, 31.7008) -> (44.4112, 31.7008)
  line L491 (42.4498, 25.0508) -> (41.6878, 25.0508)
  line L492 (36.9817, 31.3231) -> (36.6713, 31.7112)
  arc A41 (37.2921, 29.6968) -> (37.0205, 29.8132) centre (37.0205, 29.4381) ccw
  line L493 (37.2921, 26.9628) -> (37.2921, 26.6524)
  line L494 (36.6713, 24.2676) -> (37.7578, 23.9571)
  line L495 (43.4023, 32.3391) -> (44.7993, 33.1153)
  line L496 (42.4498, 26.0668) -> (41.6878, 26.0668)
  line L497 (37.2921, 21.8828) -> (37.2921, 21.4171)
  line L498 (42.7037, 29.8768) -> (42.7037, 28.8608)
  line L499 (37.7578, 22.1933) -> (37.6026, 22.1933)
  line L500 (38.0682, 31.3231) -> (38.0682, 32.0993)
  line L501 (38.0682, 26.4971) -> (38.0682, 26.8852)
  line L502 (42.4498, 32.6707) -> (41.6878, 32.6707)
  arc A42 (37.2921, 26.9628) -> (36.6713, 26.9628) centre (36.9817, 26.9628) ccw
  line L503 (38.0682, 21.4171) -> (38.0682, 21.8828)
  line L504 (42.7037, 22.2568) -> (42.7037, 21.2408)
  arc A43 (44.4112, 30.9246) -> (44.4112, 31.7008) centre (44.4112, 31.3127) ccw
  line L505 (44.4112, 30.9247) -> (43.7903, 30.9247)
  line L506 (36.6713, 26.4971) -> (36.6713, 26.9628)
  line L507 (42.4498, 22.5108) -> (41.6878, 22.5108)
  arc A44 (38.0682, 21.8828) -> (37.7578, 22.1932) centre (37.7578, 21.8828) ccw
  line L508 (37.2921, 29.6968) -> (38.0682, 29.0371)
  line L509 (37.2921, 21.4171) -> (36.6713, 21.4171)
  line L510 (44.7993, 33.1153) -> (43.4023, 33.1153)
  line L511 (42.7037, 32.4168) -> (42.7037, 31.4008)
  arc A45 (38.0683, 26.8852) -> (37.2921, 26.8852) centre (37.6802, 26.8852) ccw
  arc A46 (37.0205, 29.8133) -> (36.6712, 29.464) centre (37.0205, 29.464) ccw
  line L512 (44.7993, 32.3391) -> (43.4023, 32.3391)
  line L513 (36.6713, 31.7112) -> (38.0682, 31.7112)
  arc A47 (36.6712, 29.464) -> (36.9817, 29.0371) centre (37.1199, 29.464) ccw
  arc A48 (43.7903, 31.7008) -> (43.7903, 30.9246) centre (43.7903, 31.3127) ccw
extrude "Extrude1" add sketch "dxf" against normal blind 1.6 contours L0 L1 L2 L3 | L16 L17 A6 L21 | L30 L31 L32 L33 L35 L37 L41 L43 L45 L48 L61 L62 L78 L84 L89 L116 L121 | L36 L59 L76 L78 L81 L140 | L38 L49 L72 L79 L81 L85 L87 L115 | L59 L82 L89 L139 | L55 L76 L83 L87 | L55 L56 L57 L64 L67 L68 L70 L82 L111 L140 | L57 L116 L121 L135 L139 | L48 L58 L63 L66 L111 L135 | L49 L67 L83 L112 | A15 L85 | L47 L50 L54 L63 L65 L105 | L64 L72 L75 L112 | L51 L66 L68 L105 | L44 L47 L56 L75 L79 L137 | A11 L85 | L51 L54 L70 L137 | L85 A19 | A7 L42 L46 L71 L73 L77 | A8 L34 L39 L40 L52 L60 | A9 | A10 | L53 L100 L138 L142 | L74 L80 L99 L136 | A17 | A18 | L90 L95 L103 L133 | L91 L109 L120 L149 | L92 L93 L101 L110 | L94 L97 L128 L201 | L96 L104 L122 L144 | L98 L134 L141 L161 | L102 L123 L124 L167 | L106 L125 L127 L130 | L107 L114 L117 L126 | L108 L118 L145 L202 | L113 L131 L132 L148 | L119 L129 L170 L172 | L143 L146 L147 L154 | L150 L173 L176 L204 | L151 L153 L171 L178 | L152 L163 L181 L203 | L155 L188 L191 L209 | L156 L166 L174 L177 | L157 L175 L189 L205 | L158 L193 L196 L206 | L159 L190 L194 L199 | L160 L162 L192 L207 | L164 L187 L195 L208 | L165 L168 L169 L212 | L179 L184 L264 L269 | L180 L183 L197 L224 | L182 L210 L243 L272 | L185 L186 L211 L213 | L198 L214 L221 L251 | L200 L254 L255 L257 | L215 L241 L249 L274 L277 L278 L280 L419 L420 L432 | L217 L248 L250 L276 L288 L295 L296 L420 L429 L433 | L216 L219 L231 L281 L285 L287 L290 L291 | L216 L226 L227 L230 L247 L258 L275 L279 | L218 L222 L227 L239 L284 L286 L289 L292 | L220 L234 L242 L244 | L223 L232 L235 L266 | L225 L260 L268 L273 | L228 L229 L245 L263 | L233 L253 L256 L270 | L236 L237 L238 L267 | L240 L252 L259 L271 | L246 L261 L262 L265 | A20 | A21 A31 | L282 L297 L300 L302 L304 L319 L326 L329 L332 L336 L340 L347 | L297 L319 L329 L350 | L326 L332 L335 L340 | L283 L293 L294 L298 L439 L443 L444 L445 L446 L447 A33 A34 L459 L461 L463 L473 L475 A38 L481 A39 | L443 L445 L448 L464 L482 | L442 L444 L451 L452 L475 | L450 L459 L463 L466 L474 | L440 L441 L446 L455 L473 | A36 | A22 A26 A27 A28 A37 L484 | A23 A32 | A24 | A25 A35 | L299 L301 L307 L315 L320 L334 L345 L465 L502 L511 | L303 L305 L306 L310 L311 L339 L346 L460 L467 L491 | L308 L352 L360 L363 L386 L411 | L308 L352 L363 L369 | L308 L352 L369 L375 L412 L414 | L308 L352 L364 L412 | L308 L352 L361 L364 L377 L402 | L309 L314 L321 L327 L328 L333 L348 L458 L462 L498 | L312 L341 L344 L372 L380 L403 L406 L487 L504 L507 | L313 L323 L355 L371 L381 L407 | L313 L323 L381 L401 | L313 L323 L376 L388 L397 L401 | L313 L323 L397 L398 | L313 L323 L325 L398 L400 L415 | L316 L317 L353 L373 L384 L387 | L316 L317 L373 L392 | L316 L317 L367 L379 L392 L408 | L316 L317 L358 L408 | L316 L317 L358 L370 L378 L382 | L318 L324 L389 L396 L409 L410 | L318 L324 L410 L413 | L318 L324 L354 L368 L374 L413 | L318 L324 L354 L366 | L318 L324 L359 L366 L399 L404 | L322 L330 L331 L338 L343 L349 L351 L456 L468 L496 | A29 A30 | L337 L342 L356 L383 L391 L394 | L337 L342 L391 L393 | L337 L342 L362 L390 L393 L395 | L337 L342 L362 L385 | L337 L342 L357 L365 L385 L405 | L416 L417 L421 L437 | L418 L422 L426 L434 | L423 L454 L476 L483 | L424 L427 L453 L469 | L425 L457 L470 L480 | L428 L449 L472 L478 | L430 L431 L435 L436 | L438 L471 L477 L479 | L490 A43 L505 A48 makes body 1 in component "PCB"
extrude "Extrude2" add sketch "dxf" along normal blind 9.5 contours A7 L42 L46 L71 L73 L77 | A8 L34 L39 L40 L52 L60 bodies 1 in component "PCB"
extrude "Extrude3" add sketch "dxf" along normal blind 6 contours L282 L297 L300 L302 L304 L319 L326 L329 L332 L336 L340 L347 | L490 A43 L505 A48 bodies 1 in component "PCB"
extrude "Extrude4" add sketch "dxf" along normal blind 5 contours L299 L301 L307 L315 L320 L334 L345 L465 L502 L511 | L303 L305 L306 L310 L311 L339 L346 L460 L467 L491 | L309 L314 L321 L327 L328 L333 L348 L458 L462 L498 | L312 L341 L344 L372 L380 L403 L406 L487 L504 L507 | L322 L330 L331 L338 L343 L349 L351 L456 L468 L496 bodies 1 in component "PCB"
extrude "Extrude5" add sketch "dxf" along normal blind 6.5 contours L308 L352 L360 L363 L386 L411 | L308 L352 L363 L369 | L308 L352 L369 L375 L412 L414 | L308 L352 L364 L412 | L308 L352 L361 L364 L377 L402 | L313 L323 L355 L371 L381 L407 | L313 L323 L381 L401 | L313 L323 L376 L388 L397 L401 | L313 L323 L397 L398 | L313 L323 L325 L398 L400 L415 | L316 L317 L353 L373 L384 L387 | L316 L317 L373 L392 | L316 L317 L367 L379 L392 L408 | L316 L317 L358 L408 | L316 L317 L358 L370 L378 L382 | L318 L324 L389 L396 L409 L410 | L318 L324 L410 L413 | L318 L324 L354 L368 L374 L413 | L318 L324 L354 L366 | L318 L324 L359 L366 L399 L404 | L337 L342 L356 L383 L391 L394 | L337 L342 L391 L393 | L337 L342 L362 L390 L393 L395 | L337 L342 L362 L385 | L337 L342 L357 L365 L385 L405 bodies 1 in component "PCB"
extrude "Extrude7" add sketch "dxf" along normal blind 9.5 contours L416 L417 L421 L437 | L423 L454 L476 L483 | L424 L427 L453 L469 | L425 L457 L470 L480 | L428 L449 L472 L478 | L438 L471 L477 L479 bodies 1 in component "PCB"
extrude "Extrude6" add sketch "dxf" along normal blind 2.5 contours L216 L219 L231 L281 L285 L287 L290 L291 | L216 L226 L227 L230 L247 L258 L275 L279 | L218 L222 L227 L239 L284 L286 L289 L292 bodies 1 in component "PCB"
extrude "Extrude8" add sketch "dxf" along normal blind 9.5 contours L53 L100 L138 L142 | L74 L80 L99 L136 | L90 L95 L103 L133 | L91 L109 L120 L149 | L92 L93 L101 L110 | L94 L97 L128 L201 | L96 L104 L122 L144 | L98 L134 L141 L161 | L102 L123 L124 L167 | L106 L125 L127 L130 | L107 L114 L117 L126 | L108 L118 L145 L202 | L113 L131 L132 L148 | L119 L129 L170 L172 | L143 L146 L147 L154 | L150 L173 L176 L204 | L151 L153 L171 L178 | L152 L163 L181 L203 | L155 L188 L191 L209 | L156 L166 L174 L177 | L157 L175 L189 L205 | L158 L193 L196 L206 | L159 L190 L194 L199 | L160 L162 L192 L207 | L164 L187 L195 L208 | L165 L168 L169 L212 | L179 L184 L264 L269 | L180 L183 L197 L224 | L182 L210 L243 L272 | L185 L186 L211 L213 | L198 L214 L221 L251 | L200 L254 L255 L257 | L220 L234 L242 L244 | L223 L232 L235 L266 | L225 L260 L268 L273 | L228 L229 L245 L263 | L233 L253 L256 L270 | L236 L237 L238 L267 | L240 L252 L259 L271 | L246 L261 L262 L265 bodies 1 in component "PCB"
extrude "Extrude9" add sketch "dxf" along normal blind 2 contours L36 L59 L76 L78 L81 L140 | L55 L56 L57 L64 L67 L68 L70 L82 L111 L140 | L48 L58 L63 L66 L111 L135 | L44 L47 L56 L75 L79 L137 bodies 1 in component "PCB"
extrude "Extrude10" add sketch "dxf" along normal blind 9.5 contours L30 L31 L32 L33 L35 L37 L41 L43 L45 L48 L61 L62 L78 L84 L89 L116 L121 | L38 L49 L72 L79 L81 L85 L87 L115 | L59 L82 L89 L139 | L55 L76 L83 L87 | L57 L116 L121 L135 L139 | L49 L67 L83 L112 | A15 L85 | L47 L50 L54 L63 L65 L105 | L64 L72 L75 L112 | L51 L66 L68 L105 | A11 L85 | L51 L54 L70 L137 | L85 A19 bodies 1 in component "PCB"
extrude "Extrude11" add sketch "dxf" along normal blind 12 contours A36 bodies 1 in component "PCB"
extrude "Extrude12" add sketch "dxf" along normal blind 6.3 contours A22 A26 A27 A28 A37 L484 bodies 1 in component "PCB"
fillet "Fillet1" radius 1.2 1 edges at (38.6015, 53.4576, 12) on bodies 1 in component "PCB"
extrude "Extrude13" add sketch "dxf" along normal blind 12 contours A20 | A24 bodies 1 in component "PCB"
chamfer "Chamfer1" distance 0.25 distance2 9 1 edges at (21.3684, 64.3672, 12) measured on face at (23.482, 65.5025, 12) on bodies 1 in component "PCB"
extrude "Extrude14" add sketch "dxf" along normal blind 4 contours L283 L293 L294 L298 L439 L443 L444 L445 L446 L447 A33 A34 L459 L461 L463 L473 L475 A38 L481 A39 bodies 1 in component "PCB"
extrude "Extrude15" add sketch "dxf" along normal blind 4.5 contours A21 A31 | A23 A32 | A25 A35 | A29 A30 bodies 1 in component "PCB"
ref_plane "WorkPlane1" through (23.5, 38.5, -4.6) normal (0, 0, 1) x (1, 0, 0) in component "bottom_shell"
sketch "bottom" plane through (23.5, 38.5, -4.6) normal (0, 0, 1) x (1, 0, 0) in component "bottom_shell"
  circle A0 centre (-18.5, 33.5) radius 1.7463 construction
  circle A1 centre (18.5, 33.5) radius 1.7463 construction
  circle A2 centre (18.5, -33.5) radius 1.7463 construction
  circle A3 centre (-18.5, -33.5) radius 1.7463 construction
  line L0 (23.5, -38.5) -> (23.5, 38.5) construction
  line L1 (-23.5, -38.5) -> (23.5, -38.5) construction
  line L2 (-23.5, 38.5) -> (-23.5, -38.5) construction
  line L3 (23.5, 38.5) -> (-23.5, 38.5) construction
  line L4 (25, -39) -> (25, 39)
  line L5 (24, 40) -> (-24, 40)
  line L6 (-25, 39) -> (-25, -39)
  line L7 (-24, -40) -> (24, -40)
  arc A4 (25, 39) -> (24, 40) centre (24, 39) ccw
  arc A5 (-24, 40) -> (-25, 39) centre (-24, 39) ccw
  arc A6 (24, -40) -> (25, -39) centre (24, -39) ccw
  arc A7 (-25, -39) -> (-24, -40) centre (-24, -39) ccw
  line L8 (-25.8, 39) -> (-25.8, -39)
  arc A8 (-25.8, -39) -> (-24, -40.8) centre (-24, -39) ccw
  line L9 (-24, -40.8) -> (24, -40.8)
  arc A9 (24, -40.8) -> (25.8, -39) centre (24, -39) ccw
  line L10 (25.8, -39) -> (25.8, 39)
  arc A10 (25.8, 39) -> (24, 40.8) centre (24, 39) ccw
  line L11 (24, 40.8) -> (-24, 40.8)
  arc A11 (-24, 40.8) -> (-25.8, 39) centre (-24, 39) ccw
  line L12 (24, 42) -> (-24, 42)
  arc A12 (-24, 42) -> (-27, 39) centre (-24, 39) ccw
  line L13 (-27, 39) -> (-27, -39)
  arc A13 (-27, -39) -> (-24, -42) centre (-24, -39) ccw
  line L14 (-24, -42) -> (24, -42)
  arc A14 (24, -42) -> (27, -39) centre (24, -39) ccw
  line L15 (27, -39) -> (27, 39)
  arc A15 (27, 39) -> (24, 42) centre (24, 39) ccw
  circle A16 centre (-18.5, 33.5) radius 1.75
  circle A17 centre (-18.5, 33.5) radius 3
  circle A18 centre (-18.5, 33.5) radius 5
  circle A19 centre (-18.5, -33.5) radius 1.75
  circle A20 centre (-18.5, -33.5) radius 3
  circle A21 centre (-18.5, -33.5) radius 5
  circle A22 centre (18.5, -33.5) radius 5
  circle A23 centre (18.5, -33.5) radius 3
  circle A24 centre (18.5, -33.5) radius 1.75
  circle A25 centre (18.5, 33.5) radius 1.75
  circle A26 centre (18.5, 33.5) radius 3
  circle A27 centre (18.5, 33.5) radius 5
  dimension "d42" = 1
  dimension "d43" = 0.8
  dimension "d44" = 2
  dimension "d48" = 3.5
  dimension "d49" = 6
  dimension "d50" = 10
  dimension "d51" = 3.5
  dimension "d52" = 6
  dimension "d53" = 10
  dimension "d54" = 10
  dimension "d55" = 6
  dimension "d56" = 3.5
  dimension "d57" = 3.5
  dimension "d58" = 6
  dimension "d59" = 10
  constraint parallel L0 L4
  constraint parallel L3 L5
  constraint parallel L2 L6
  constraint parallel L1 L7
  constraint tangent L4 A4
  constraint tangent L5 A4
  constraint tangent L5 A5
  constraint tangent L6 A5
  constraint equal A4 A5
  constraint tangent L4 A6
  constraint tangent L7 A6
  constraint equal A4 A6
  constraint tangent L6 A7
  constraint tangent L7 A7
  constraint equal A4 A7
  constraint concentric A0 A16
  constraint concentric A0 A17
  constraint concentric A17 A18
  constraint concentric A3 A19
  constraint concentric A19 A20
  constraint concentric A19 A21
  constraint concentric A2 A22
  constraint concentric A22 A23
  constraint concentric A23 A24
  constraint concentric A1 A25
  constraint concentric A1 A26
  constraint concentric A25 A27
  measures "d42" radius of A4
  measures "d48" diameter of A16
  measures "d49" diameter of A17
  measures "d50" diameter of A18
  measures "d51" diameter of A19
  measures "d52" diameter of A20
  measures "d53" diameter of A21
  measures "d54" diameter of A22
  measures "d55" diameter of A23
  measures "d56" diameter of A24
  measures "d57" diameter of A25
  measures "d58" diameter of A26
  measures "d59" diameter of A27
extrude "Extrude1'" add sketch "bottom" against normal blind 2 separate body contours L4 L5 L6 L7 A4 A5 A6 A7 | L8 A8 L9 A9 L10 A10 L11 A11 | L12 A12 L13 A13 L14 A14 L15 A15 | A18 | A21 | A22 | A27 makes body 2 in component "bottom_shell"
extrude "Extrude2'" add sketch "bottom" along normal blind 3 contours A17 | A18 | A20 | A21 | A22 | A23 | A26 | A27 bodies 2 in component "bottom_shell"
chamfer "Chamfer1'" distance 2 distance2 2 4 edges at (37.3384, 3.1919, -1.6) (0.3384, 3.1919, -1.6) (0.3384, 70.1919, -1.6) (37.3384, 70.1919, -1.6) measured on face at (45.8915, 4.6647, -1.6) measured on face at (8.8915, 4.6647, -1.6) measured on face at (8.8981, 71.7516, -1.6) measured on face at (45.8981, 71.7516, -1.6) on bodies 2 in component "bottom_shell"
extrude "Extrude3'" add sketch "bottom" along normal blind 11.1 contours L12 A12 L13 A13 L14 A14 L15 A15 bodies 2 in component "bottom_shell"
extrude "Extrude4'" add sketch "bottom" along normal blind 12.6 contours L8 A8 L9 A9 L10 A10 L11 A11 bodies 2 in component "bottom_shell"
fillet "Fillet1'" radius 2 8 edges at (23.5, -3.5, -6.6) (-2.6213, -2.6213, -6.6) (-3.5, 38.5, -6.6) (-2.6213, 79.6213, -6.6) (23.5, 80.5, -6.6) (49.6213, 79.6213, -6.6) (50.5, 38.5, -6.6) (49.6213, -2.6213, -6.6) on bodies 2 in component "bottom_shell"
fillet "Fillet2" radius 0.5 12 edges at (23.5, 78.5, -4.6) (-1.2071, 78.2071, -4.6) (-1.5, 38.5, -4.6) (-1.2071, -1.2071, -4.6) (23.5, -1.5, -4.6) (48.2071, -1.2071, -4.6) (48.5, 38.5, -4.6) (48.2071, 78.2071, -4.6) (37.3384, 73.8081, -4.6) (37.3384, 6.8081, -4.6) (0.3384, 73.8081, -4.6) (0.3384, 6.8081, -4.6) on bodies 2 in component "bottom_shell"
ref_plane "WorkPlane1" through (0, 0, 9) normal (0, 0, 1) x (1, 0, 0) in component "top_shell"